Autodesk Fusion 360 part; units mm, degrees
(part 2 of 3)
sketch "Sketch6" plane through (0, 0, 6) normal (0, 0, 1) x (1, 0, 0)
  arc A0 (8.0454, -2.2316) -> (8.0834, -2.0901) centre (0, 0) ccw
  arc A1 (9.1959, -1.3509) -> (8.0834, -2.0901) centre (9.0515, -2.3404) ccw
  line L0 (9.1959, -1.3509) -> (9.7621, -1.4335)
  spline S0 degree 5 poles (9.7621, -1.4335) (9.7691, -1.4345) (9.783, -1.4364) (9.8041, -1.4384) (9.8322, -1.4399) (9.8676, -1.44) (9.903, -1.4389) (9.9385, -1.437) (9.9741, -1.4347) (10.0097, -1.4321) (10.0453, -1.4292) (10.081, -1.4258) (10.1167, -1.422) (10.1525, -1.4175) (10.1882, -1.4124) (10.224, -1.4067) (10.2599, -1.4005) (10.2957, -1.3939) (10.3316, -1.387) (10.3674, -1.3797) (10.4033, -1.3721) (10.4391, -1.364) (10.475, -1.3556) (10.5109, -1.3469) (10.5468, -1.3377) (10.5826, -1.3281) (10.6185, -1.3182) (10.6543, -1.3079) (10.6902, -1.2973) (10.726, -1.2864) (10.7619, -1.2752) (10.7977, -1.2636) (10.8335, -1.2517) (10.8693, -1.2395) (10.905, -1.227) (10.9408, -1.2141) (10.9765, -1.2009) (11.0122, -1.1875) (11.0479, -1.1737) (11.0835, -1.1597) (11.1191, -1.1453) (11.1547, -1.1307) (11.1903, -1.1158) (11.2259, -1.1005) (11.2614, -1.085) (11.2968, -1.0692) (11.3323, -1.0532) (11.3677, -1.0368) (11.4031, -1.0202) (11.4384, -1.0033) (11.4737, -0.9861) (11.5089, -0.9687) (11.5441, -0.951) (11.5793, -0.933) (11.6144, -0.9148) (11.6495, -0.8963) (11.6845, -0.8775) (11.7195, -0.8585) (11.7545, -0.8392) (11.7894, -0.8197) (11.8242, -0.7999) (11.859, -0.7799) (11.8937, -0.7596) (11.9284, -0.7391) (11.963, -0.7183) (11.9976, -0.6972) (12.0321, -0.6759) (12.0666, -0.6544) (12.101, -0.6327) (12.1353, -0.6106) (12.1696, -0.5884) (12.197, -0.5704) (12.2175, -0.5568) (12.2311, -0.5477) (12.238, -0.5431) knots 0 0 0 0 0 0 0.01428571 0.02857143 0.04285714 0.05714286 0.07142857 0.08571429 0.1 0.11428571 0.12857143 0.14285714 0.15714286 0.17142857 0.18571429 0.2 0.21428571 0.22857143 0.24285714 0.25714286 0.27142857 0.28571429 0.3 0.31428571 0.32857143 0.34285714 0.35714286 0.37142857 0.38571429 0.4 0.41428571 0.42857143 0.44285714 0.45714286 0.47142857 0.48571429 0.5 0.51428571 0.52857143 0.54285714 0.55714286 0.57142857 0.58571429 0.6 0.61428571 0.62857143 0.64285714 0.65714286 0.67142857 0.68571429 0.7 0.71428571 0.72857143 0.74285714 0.75714286 0.77142857 0.78571429 0.8 0.81428571 0.82857143 0.84285714 0.85714286 0.87142857 0.88571429 0.9 0.91428571 0.92857143 0.94285714 0.95714286 0.97142857 0.98571429 1 1 1 1 1 1
  arc A2 (12.238, -0.5431) -> (12.238, 0.5431) centre (0, 0) ccw
  spline S1 degree 5 poles (12.238, 0.5431) (12.2311, 0.5477) (12.2175, 0.5568) (12.197, 0.5704) (12.1696, 0.5884) (12.1353, 0.6106) (12.101, 0.6327) (12.0666, 0.6544) (12.0321, 0.6759) (11.9976, 0.6972) (11.963, 0.7183) (11.9284, 0.7391) (11.8937, 0.7596) (11.859, 0.7799) (11.8242, 0.7999) (11.7894, 0.8197) (11.7545, 0.8392) (11.7195, 0.8585) (11.6845, 0.8775) (11.6495, 0.8963) (11.6144, 0.9148) (11.5793, 0.933) (11.5441, 0.951) (11.5089, 0.9687) (11.4737, 0.9861) (11.4384, 1.0033) (11.4031, 1.0202) (11.3677, 1.0368) (11.3323, 1.0532) (11.2968, 1.0692) (11.2614, 1.085) (11.2259, 1.1005) (11.1903, 1.1158) (11.1547, 1.1307) (11.1191, 1.1453) (11.0835, 1.1597) (11.0479, 1.1737) (11.0122, 1.1875) (10.9765, 1.2009) (10.9408, 1.2141) (10.905, 1.227) (10.8693, 1.2395) (10.8335, 1.2517) (10.7977, 1.2636) (10.7619, 1.2752) (10.726, 1.2864) (10.6902, 1.2973) (10.6543, 1.3079) (10.6185, 1.3182) (10.5826, 1.3281) (10.5468, 1.3377) (10.5109, 1.3469) (10.475, 1.3556) (10.4391, 1.364) (10.4033, 1.3721) (10.3674, 1.3797) (10.3316, 1.387) (10.2957, 1.3939) (10.2599, 1.4005) (10.224, 1.4067) (10.1882, 1.4124) (10.1525, 1.4175) (10.1167, 1.422) (10.081, 1.4258) (10.0453, 1.4292) (10.0097, 1.4321) (9.9741, 1.4347) (9.9385, 1.437) (9.903, 1.4389) (9.8676, 1.44) (9.8322, 1.4399) (9.8041, 1.4384) (9.783, 1.4364) (9.7691, 1.4345) (9.7621, 1.4335) knots -1 -1 -1 -1 -1 -1 -0.98571429 -0.97142857 -0.95714286 -0.94285714 -0.92857143 -0.91428571 -0.9 -0.88571429 -0.87142857 -0.85714286 -0.84285714 -0.82857143 -0.81428571 -0.8 -0.78571429 -0.77142857 -0.75714286 -0.74285714 -0.72857143 -0.71428571 -0.7 -0.68571429 -0.67142857 -0.65714286 -0.64285714 -0.62857143 -0.61428571 -0.6 -0.58571429 -0.57142857 -0.55714286 -0.54285714 -0.52857143 -0.51428571 -0.5 -0.48571429 -0.47142857 -0.45714286 -0.44285714 -0.42857143 -0.41428571 -0.4 -0.38571429 -0.37142857 -0.35714286 -0.34285714 -0.32857143 -0.31428571 -0.3 -0.28571429 -0.27142857 -0.25714286 -0.24285714 -0.22857143 -0.21428571 -0.2 -0.18571429 -0.17142857 -0.15714286 -0.14285714 -0.12857143 -0.11428571 -0.1 -0.08571429 -0.07142857 -0.05714286 -0.04285714 -0.02857143 -0.01428571 0 0 0 0 0 0
  line L1 (9.7621, 1.4335) -> (9.1959, 1.3509)
  arc A3 (8.0834, 2.0901) -> (9.1959, 1.3509) centre (9.0515, 2.3404) ccw
  arc A4 (8.0834, 2.0901) -> (8.0454, 2.2316) centre (0, 0) ccw
  arc A5 (8.6393, 3.428) -> (8.0454, 2.2316) centre (9.0091, 2.4989) ccw
  line L2 (8.6393, 3.428) -> (9.171, 3.6396)
  spline S2 degree 5 poles (9.171, 3.6396) (9.1775, 3.6422) (9.1905, 3.6476) (9.2098, 3.6563) (9.2349, 3.6691) (9.2656, 3.6867) (9.2957, 3.7054) (9.3255, 3.7248) (9.3552, 3.7446) (9.3847, 3.7646) (9.4141, 3.785) (9.4433, 3.8057) (9.4723, 3.8269) (9.501, 3.8487) (9.5295, 3.871) (9.5576, 3.8938) (9.5856, 3.917) (9.6133, 3.9407) (9.6409, 3.9646) (9.6683, 3.9888) (9.6955, 4.0134) (9.7226, 4.0383) (9.7494, 4.0635) (9.7761, 4.089) (9.8026, 4.1149) (9.8289, 4.1411) (9.855, 4.1677) (9.8809, 4.1945) (9.9066, 4.2216) (9.9322, 4.249) (9.9576, 4.2766) (9.9829, 4.3045) (10.0079, 4.3327) (10.0328, 4.3612) (10.0575, 4.3899) (10.082, 4.4189) (10.1064, 4.4482) (10.1306, 4.4777) (10.1546, 4.5075) (10.1785, 4.5375) (10.2021, 4.5677) (10.2256, 4.5982) (10.249, 4.6289) (10.2721, 4.6598) (10.2951, 4.691) (10.318, 4.7224) (10.3406, 4.7541) (10.3631, 4.7859) (10.3854, 4.818) (10.4076, 4.8503) (10.4296, 4.8828) (10.4514, 4.9155) (10.473, 4.9485) (10.4945, 4.9816) (10.5158, 5.015) (10.5369, 5.0485) (10.5579, 5.0823) (10.5787, 5.1163) (10.5993, 5.1504) (10.6197, 5.1848) (10.64, 5.2193) (10.6601, 5.2541) (10.6801, 5.289) (10.6998, 5.3242) (10.7194, 5.3595) (10.7388, 5.395) (10.7581, 5.4307) (10.7772, 5.4665) (10.7961, 5.5026) (10.8148, 5.5388) (10.8334, 5.5752) (10.8481, 5.6045) (10.859, 5.6265) (10.8663, 5.6413) (10.8699, 5.6486) knots 0 0 0 0 0 0 0.01428571 0.02857143 0.04285714 0.05714286 0.07142857 0.08571429 0.1 0.11428571 0.12857143 0.14285714 0.15714286 0.17142857 0.18571429 0.2 0.21428571 0.22857143 0.24285714 0.25714286 0.27142857 0.28571429 0.3 0.31428571 0.32857143 0.34285714 0.35714286 0.37142857 0.38571429 0.4 0.41428571 0.42857143 0.44285714 0.45714286 0.47142857 0.48571429 0.5 0.51428571 0.52857143 0.54285714 0.55714286 0.57142857 0.58571429 0.6 0.61428571 0.62857143 0.64285714 0.65714286 0.67142857 0.68571429 0.7 0.71428571 0.72857143 0.74285714 0.75714286 0.77142857 0.78571429 0.8 0.81428571 0.82857143 0.84285714 0.85714286 0.87142857 0.88571429 0.9 0.91428571 0.92857143 0.94285714 0.95714286 0.97142857 0.98571429 1 1 1 1 1 1
  arc A6 (10.8699, 5.6486) -> (10.3268, 6.5893) centre (0, 0) ccw
  spline S3 degree 5 poles (10.3268, 6.5893) (10.3186, 6.5899) (10.3022, 6.5909) (10.2777, 6.5925) (10.245, 6.5944) (10.2042, 6.5965) (10.1634, 6.5984) (10.1228, 6.6) (10.0821, 6.6014) (10.0416, 6.6026) (10.0012, 6.6036) (9.9608, 6.6042) (9.9205, 6.6047) (9.8802, 6.6049) (9.8401, 6.6049) (9.8, 6.6046) (9.76, 6.604) (9.7202, 6.6033) (9.6803, 6.6022) (9.6406, 6.601) (9.601, 6.5994) (9.5615, 6.5977) (9.522, 6.5957) (9.4827, 6.5934) (9.4434, 6.5909) (9.4043, 6.5881) (9.3652, 6.585) (9.3263, 6.5818) (9.2875, 6.5782) (9.2487, 6.5744) (9.2101, 6.5703) (9.1716, 6.566) (9.1332, 6.5614) (9.095, 6.5566) (9.0568, 6.5515) (9.0188, 6.5461) (8.9809, 6.5404) (8.9431, 6.5345) (8.9054, 6.5283) (8.8679, 6.5218) (8.8305, 6.5151) (8.7933, 6.5081) (8.7562, 6.5007) (8.7193, 6.4931) (8.6825, 6.4852) (8.6458, 6.4771) (8.6093, 6.4686) (8.573, 6.4599) (8.5368, 6.4508) (8.5008, 6.4415) (8.4649, 6.4318) (8.4293, 6.4218) (8.3938, 6.4115) (8.3585, 6.4009) (8.3235, 6.3899) (8.2886, 6.3786) (8.2539, 6.367) (8.2194, 6.355) (8.185, 6.3428) (8.1509, 6.3303) (8.1171, 6.3173) (8.0836, 6.3038) (8.0504, 6.2898) (8.0175, 6.2753) (7.9849, 6.2604) (7.9526, 6.2451) (7.9205, 6.2295) (7.8885, 6.2138) (7.8568, 6.1976) (7.8255, 6.1809) (7.795, 6.1631) (7.7714, 6.1477) (7.7542, 6.1354) (7.743, 6.1269) (7.7374, 6.1225) knots -1 -1 -1 -1 -1 -1 -0.98571429 -0.97142857 -0.95714286 -0.94285714 -0.92857143 -0.91428571 -0.9 -0.88571429 -0.87142857 -0.85714286 -0.84285714 -0.82857143 -0.81428571 -0.8 -0.78571429 -0.77142857 -0.75714286 -0.74285714 -0.72857143 -0.71428571 -0.7 -0.68571429 -0.67142857 -0.65714286 -0.64285714 -0.62857143 -0.61428571 -0.6 -0.58571429 -0.57142857 -0.55714286 -0.54285714 -0.52857143 -0.51428571 -0.5 -0.48571429 -0.47142857 -0.45714286 -0.44285714 -0.42857143 -0.41428571 -0.4 -0.38571429 -0.37142857 -0.35714286 -0.34285714 -0.32857143 -0.31428571 -0.3 -0.28571429 -0.27142857 -0.25714286 -0.24285714 -0.22857143 -0.21428571 -0.2 -0.18571429 -0.17142857 -0.15714286 -0.14285714 -0.12857143 -0.11428571 -0.1 -0.08571429 -0.07142857 -0.05714286 -0.04285714 -0.02857143 -0.01428571 0 0 0 0 0 0
  line L3 (7.7374, 6.1225) -> (7.2884, 5.7679)
  arc A7 (5.9553, 5.8518) -> (7.2884, 5.7679) centre (6.6686, 6.5526) ccw
  arc A8 (5.9553, 5.8518) -> (5.8518, 5.9553) centre (0, 0) ccw
  arc A9 (5.7679, 7.2884) -> (5.8518, 5.9553) centre (6.5526, 6.6686) ccw
  line L4 (5.7679, 7.2884) -> (6.1225, 7.7374)
  spline S4 degree 5 poles (6.1225, 7.7374) (6.1269, 7.743) (6.1354, 7.7542) (6.1477, 7.7714) (6.1631, 7.795) (6.1809, 7.8255) (6.1976, 7.8568) (6.2138, 7.8885) (6.2295, 7.9205) (6.2451, 7.9526) (6.2604, 7.9849) (6.2753, 8.0175) (6.2898, 8.0504) (6.3038, 8.0836) (6.3173, 8.1171) (6.3303, 8.1509) (6.3428, 8.185) (6.355, 8.2194) (6.367, 8.2539) (6.3786, 8.2886) (6.3899, 8.3235) (6.4009, 8.3585) (6.4115, 8.3938) (6.4218, 8.4293) (6.4318, 8.4649) (6.4415, 8.5008) (6.4508, 8.5368) (6.4599, 8.573) (6.4686, 8.6093) (6.4771, 8.6458) (6.4852, 8.6825) (6.4931, 8.7193) (6.5007, 8.7562) (6.5081, 8.7933) (6.5151, 8.8305) (6.5218, 8.8679) (6.5283, 8.9054) (6.5345, 8.9431) (6.5404, 8.9809) (6.5461, 9.0188) (6.5515, 9.0568) (6.5566, 9.095) (6.5614, 9.1332) (6.566, 9.1716) (6.5703, 9.2101) (6.5744, 9.2487) (6.5782, 9.2875) (6.5818, 9.3263) (6.585, 9.3652) (6.5881, 9.4043) (6.5909, 9.4434) (6.5934, 9.4827) (6.5957, 9.522) (6.5977, 9.5615) (6.5994, 9.601) (6.601, 9.6406) (6.6022, 9.6803) (6.6033, 9.7202) (6.604, 9.76) (6.6046, 9.8) (6.6049, 9.8401) (6.6049, 9.8802) (6.6047, 9.9205) (6.6042, 9.9608) (6.6036, 10.0012) (6.6026, 10.0416) (6.6014, 10.0821) (6.6, 10.1228) (6.5984, 10.1634) (6.5965, 10.2042) (6.5944, 10.245) (6.5925, 10.2777) (6.5909, 10.3022) (6.5899, 10.3186) (6.5893, 10.3268) knots 0 0 0 0 0 0 0.01428571 0.02857143 0.04285714 0.05714286 0.07142857 0.08571429 0.1 0.11428571 0.12857143 0.14285714 0.15714286 0.17142857 0.18571429 0.2 0.21428571 0.22857143 0.24285714 0.25714286 0.27142857 0.28571429 0.3 0.31428571 0.32857143 0.34285714 0.35714286 0.37142857 0.38571429 0.4 0.41428571 0.42857143 0.44285714 0.45714286 0.47142857 0.48571429 0.5 0.51428571 0.52857143 0.54285714 0.55714286 0.57142857 0.58571429 0.6 0.61428571 0.62857143 0.64285714 0.65714286 0.67142857 0.68571429 0.7 0.71428571 0.72857143 0.74285714 0.75714286 0.77142857 0.78571429 0.8 0.81428571 0.82857143 0.84285714 0.85714286 0.87142857 0.88571429 0.9 0.91428571 0.92857143 0.94285714 0.95714286 0.97142857 0.98571429 1 1 1 1 1 1
  arc A10 (6.5893, 10.3268) -> (5.6486, 10.8699) centre (0, 0) ccw
  spline S5 degree 5 poles (5.6486, 10.8699) (5.6413, 10.8663) (5.6265, 10.859) (5.6045, 10.8481) (5.5752, 10.8334) (5.5388, 10.8148) (5.5026, 10.7961) (5.4665, 10.7772) (5.4307, 10.7581) (5.395, 10.7388) (5.3595, 10.7194) (5.3242, 10.6998) (5.289, 10.6801) (5.2541, 10.6601) (5.2193, 10.64) (5.1848, 10.6197) (5.1504, 10.5993) (5.1163, 10.5787) (5.0823, 10.5579) (5.0485, 10.5369) (5.015, 10.5158) (4.9816, 10.4945) (4.9485, 10.473) (4.9155, 10.4514) (4.8828, 10.4296) (4.8503, 10.4076) (4.818, 10.3854) (4.7859, 10.3631) (4.7541, 10.3406) (4.7224, 10.318) (4.691, 10.2951) (4.6598, 10.2721) (4.6289, 10.249) (4.5982, 10.2256) (4.5677, 10.2021) (4.5375, 10.1785) (4.5075, 10.1546) (4.4777, 10.1306) (4.4482, 10.1064) (4.4189, 10.082) (4.3899, 10.0575) (4.3612, 10.0328) (4.3327, 10.0079) (4.3045, 9.9829) (4.2766, 9.9576) (4.249, 9.9322) (4.2216, 9.9066) (4.1945, 9.8809) (4.1677, 9.855) (4.1411, 9.8289) (4.1149, 9.8026) (4.089, 9.7761) (4.0635, 9.7494) (4.0383, 9.7226) (4.0134, 9.6955) (3.9888, 9.6683) (3.9646, 9.6409) (3.9407, 9.6133) (3.917, 9.5856) (3.8938, 9.5576) (3.871, 9.5295) (3.8487, 9.501) (3.8269, 9.4723) (3.8057, 9.4433) (3.785, 9.4141) (3.7646, 9.3847) (3.7446, 9.3552) (3.7248, 9.3255) (3.7054, 9.2957) (3.6867, 9.2656) (3.6691, 9.2349) (3.6563, 9.2098) (3.6476, 9.1905) (3.6422, 9.1775) (3.6396, 9.171) knots -1 -1 -1 -1 -1 -1 -0.98571429 -0.97142857 -0.95714286 -0.94285714 -0.92857143 -0.91428571 -0.9 -0.88571429 -0.87142857 -0.85714286 -0.84285714 -0.82857143 -0.81428571 -0.8 -0.78571429 -0.77142857 -0.75714286 -0.74285714 -0.72857143 -0.71428571 -0.7 -0.68571429 -0.67142857 -0.65714286 -0.64285714 -0.62857143 -0.61428571 -0.6 -0.58571429 -0.57142857 -0.55714286 -0.54285714 -0.52857143 -0.51428571 -0.5 -0.48571429 -0.47142857 -0.45714286 -0.44285714 -0.42857143 -0.41428571 -0.4 -0.38571429 -0.37142857 -0.35714286 -0.34285714 -0.32857143 -0.31428571 -0.3 -0.28571429 -0.27142857 -0.25714286 -0.24285714 -0.22857143 -0.21428571 -0.2 -0.18571429 -0.17142857 -0.15714286 -0.14285714 -0.12857143 -0.11428571 -0.1 -0.08571429 -0.07142857 -0.05714286 -0.04285714 -0.02857143 -0.01428571 0 0 0 0 0 0
  line L5 (3.6396, 9.171) -> (3.428, 8.6393)
  arc A11 (2.2316, 8.0454) -> (3.428, 8.6393) centre (2.4989, 9.0091) ccw
  arc A12 (2.2316, 8.0454) -> (2.0901, 8.0834) centre (0, 0) ccw
  arc A13 (1.3509, 9.1959) -> (2.0901, 8.0834) centre (2.3404, 9.0515) ccw
  line L6 (1.3509, 9.1959) -> (1.4335, 9.7621)
  spline S6 degree 5 poles (1.4335, 9.7621) (1.4345, 9.7691) (1.4364, 9.783) (1.4384, 9.8041) (1.4399, 9.8322) (1.44, 9.8676) (1.4389, 9.903) (1.437, 9.9385) (1.4347, 9.9741) (1.4321, 10.0097) (1.4292, 10.0453) (1.4258, 10.081) (1.422, 10.1167) (1.4175, 10.1525) (1.4124, 10.1882) (1.4067, 10.224) (1.4005, 10.2599) (1.3939, 10.2957) (1.387, 10.3316) (1.3797, 10.3674) (1.3721, 10.4033) (1.364, 10.4391) (1.3556, 10.475) (1.3469, 10.5109) (1.3377, 10.5468) (1.3281, 10.5826) (1.3182, 10.6185) (1.3079, 10.6543) (1.2973, 10.6902) (1.2864, 10.726) (1.2752, 10.7619) (1.2636, 10.7977) (1.2517, 10.8335) (1.2395, 10.8693) (1.227, 10.905) (1.2141, 10.9408) (1.2009, 10.9765) (1.1875, 11.0122) (1.1737, 11.0479) (1.1597, 11.0835) (1.1453, 11.1191) (1.1307, 11.1547) (1.1158, 11.1903) (1.1005, 11.2259) (1.085, 11.2614) (1.0692, 11.2968) (1.0532, 11.3323) (1.0368, 11.3677) (1.0202, 11.4031) (1.0033, 11.4384) (0.9861, 11.4737) (0.9687, 11.5089) (0.951, 11.5441) (0.933, 11.5793) (0.9148, 11.6144) (0.8963, 11.6495) (0.8775, 11.6845) (0.8585, 11.7195) (0.8392, 11.7545) (0.8197, 11.7894) (0.7999, 11.8242) (0.7799, 11.859) (0.7596, 11.8937) (0.7391, 11.9284) (0.7183, 11.963) (0.6972, 11.9976) (0.6759, 12.0321) (0.6544, 12.0666) (0.6327, 12.101) (0.6106, 12.1353) (0.5884, 12.1696) (0.5704, 12.197) (0.5568, 12.2175) (0.5477, 12.2311) (0.5431, 12.238) knots 0 0 0 0 0 0 0.01428571 0.02857143 0.04285714 0.05714286 0.07142857 0.08571429 0.1 0.11428571 0.12857143 0.14285714 0.15714286 0.17142857 0.18571429 0.2 0.21428571 0.22857143 0.24285714 0.25714286 0.27142857 0.28571429 0.3 0.31428571 0.32857143 0.34285714 0.35714286 0.37142857 0.38571429 0.4 0.41428571 0.42857143 0.44285714 0.45714286 0.47142857 0.48571429 0.5 0.51428571 0.52857143 0.54285714 0.55714286 0.57142857 0.58571429 0.6 0.61428571 0.62857143 0.64285714 0.65714286 0.67142857 0.68571429 0.7 0.71428571 0.72857143 0.74285714 0.75714286 0.77142857 0.78571429 0.8 0.81428571 0.82857143 0.84285714 0.85714286 0.87142857 0.88571429 0.9 0.91428571 0.92857143 0.94285714 0.95714286 0.97142857 0.98571429 1 1 1 1 1 1
  arc A14 (0.5431, 12.238) -> (-0.5431, 12.238) centre (0, 0) ccw
  spline S7 degree 5 poles (-0.5431, 12.238) (-0.5477, 12.2311) (-0.5568, 12.2175) (-0.5704, 12.197) (-0.5884, 12.1696) (-0.6106, 12.1353) (-0.6327, 12.101) (-0.6544, 12.0666) (-0.6759, 12.0321) (-0.6972, 11.9976) (-0.7183, 11.963) (-0.7391, 11.9284) (-0.7596, 11.8937) (-0.7799, 11.859) (-0.7999, 11.8242) (-0.8197, 11.7894) (-0.8392, 11.7545) (-0.8585, 11.7195) (-0.8775, 11.6845) (-0.8963, 11.6495) (-0.9148, 11.6144) (-0.933, 11.5793) (-0.951, 11.5441) (-0.9687, 11.5089) (-0.9861, 11.4737) (-1.0033, 11.4384) (-1.0202, 11.4031) (-1.0368, 11.3677) (-1.0532, 11.3323) (-1.0692, 11.2968) (-1.085, 11.2614) (-1.1005, 11.2259) (-1.1158, 11.1903) (-1.1307, 11.1547) (-1.1453, 11.1191) (-1.1597, 11.0835) (-1.1737, 11.0479) (-1.1875, 11.0122) (-1.2009, 10.9765) (-1.2141, 10.9408) (-1.227, 10.905) (-1.2395, 10.8693) (-1.2517, 10.8335) (-1.2636, 10.7977) (-1.2752, 10.7619) (-1.2864, 10.726) (-1.2973, 10.6902) (-1.3079, 10.6543) (-1.3182, 10.6185) (-1.3281, 10.5826) (-1.3377, 10.5468) (-1.3469, 10.5109) (-1.3556, 10.475) (-1.364, 10.4391) (-1.3721, 10.4033) (-1.3797, 10.3674) (-1.387, 10.3316) (-1.3939, 10.2957) (-1.4005, 10.2599) (-1.4067, 10.224) (-1.4124, 10.1882) (-1.4175, 10.1525) (-1.422, 10.1167) (-1.4258, 10.081) (-1.4292, 10.0453) (-1.4321, 10.0097) (-1.4347, 9.9741) (-1.437, 9.9385) (-1.4389, 9.903) (-1.44, 9.8676) (-1.4399, 9.8322) (-1.4384, 9.8041) (-1.4364, 9.783) (-1.4345, 9.7691) (-1.4335, 9.7621) knots -1 -1 -1 -1 -1 -1 -0.98571429 -0.97142857 -0.95714286 -0.94285714 -0.92857143 -0.91428571 -0.9 -0.88571429 -0.87142857 -0.85714286 -0.84285714 -0.82857143 -0.81428571 -0.8 -0.78571429 -0.77142857 -0.75714286 -0.74285714 -0.72857143 -0.71428571 -0.7 -0.68571429 -0.67142857 -0.65714286 -0.64285714 -0.62857143 -0.61428571 -0.6 -0.58571429 -0.57142857 -0.55714286 -0.54285714 -0.52857143 -0.51428571 -0.5 -0.48571429 -0.47142857 -0.45714286 -0.44285714 -0.42857143 -0.41428571 -0.4 -0.38571429 -0.37142857 -0.35714286 -0.34285714 -0.32857143 -0.31428571 -0.3 -0.28571429 -0.27142857 -0.25714286 -0.24285714 -0.22857143 -0.21428571 -0.2 -0.18571429 -0.17142857 -0.15714286 -0.14285714 -0.12857143 -0.11428571 -0.1 -0.08571429 -0.07142857 -0.05714286 -0.04285714 -0.02857143 -0.01428571 0 0 0 0 0 0
  line L7 (-1.4335, 9.7621) -> (-1.3509, 9.1959)
  arc A15 (-2.0901, 8.0834) -> (-1.3509, 9.1959) centre (-2.3404, 9.0515) ccw
  arc A16 (-2.0901, 8.0834) -> (-2.2316, 8.0454) centre (0, 0) ccw
  arc A17 (-3.428, 8.6393) -> (-2.2316, 8.0454) centre (-2.4989, 9.0091) ccw
  line L8 (-3.428, 8.6393) -> (-3.6396, 9.171)
  spline S8 degree 5 poles (-3.6396, 9.171) (-3.6422, 9.1775) (-3.6476, 9.1905) (-3.6563, 9.2098) (-3.6691, 9.2349) (-3.6867, 9.2656) (-3.7054, 9.2957) (-3.7248, 9.3255) (-3.7446, 9.3552) (-3.7646, 9.3847) (-3.785, 9.4141) (-3.8057, 9.4433) (-3.8269, 9.4723) (-3.8487, 9.501) (-3.871, 9.5295) (-3.8938, 9.5576) (-3.917, 9.5856) (-3.9407, 9.6133) (-3.9646, 9.6409) (-3.9888, 9.6683) (-4.0134, 9.6955) (-4.0383, 9.7226) (-4.0635, 9.7494) (-4.089, 9.7761) (-4.1149, 9.8026) (-4.1411, 9.8289) (-4.1677, 9.855) (-4.1945, 9.8809) (-4.2216, 9.9066) (-4.249, 9.9322) (-4.2766, 9.9576) (-4.3045, 9.9829) (-4.3327, 10.0079) (-4.3612, 10.0328) (-4.3899, 10.0575) (-4.4189, 10.082) (-4.4482, 10.1064) (-4.4777, 10.1306) (-4.5075, 10.1546) (-4.5375, 10.1785) (-4.5677, 10.2021) (-4.5982, 10.2256) (-4.6289, 10.249) (-4.6598, 10.2721) (-4.691, 10.2951) (-4.7224, 10.318) (-4.7541, 10.3406) (-4.7859, 10.3631) (-4.818, 10.3854) (-4.8503, 10.4076) (-4.8828, 10.4296) (-4.9155, 10.4514) (-4.9485, 10.473) (-4.9816, 10.4945) (-5.015, 10.5158) (-5.0485, 10.5369) (-5.0823, 10.5579) (-5.1163, 10.5787) (-5.1504, 10.5993) (-5.1848, 10.6197) (-5.2193, 10.64) (-5.2541, 10.6601) (-5.289, 10.6801) (-5.3242, 10.6998) (-5.3595, 10.7194) (-5.395, 10.7388) (-5.4307, 10.7581) (-5.4665, 10.7772) (-5.5026, 10.7961) (-5.5388, 10.8148) (-5.5752, 10.8334) (-5.6045, 10.8481) (-5.6265, 10.859) (-5.6413, 10.8663) (-5.6486, 10.8699) knots 0 0 0 0 0 0 0.01428571 0.02857143 0.04285714 0.05714286 0.07142857 0.08571429 0.1 0.11428571 0.12857143 0.14285714 0.15714286 0.17142857 0.18571429 0.2 0.21428571 0.22857143 0.24285714 0.25714286 0.27142857 0.28571429 0.3 0.31428571 0.32857143 0.34285714 0.35714286 0.37142857 0.38571429 0.4 0.41428571 0.42857143 0.44285714 0.45714286 0.47142857 0.48571429 0.5 0.51428571 0.52857143 0.54285714 0.55714286 0.57142857 0.58571429 0.6 0.61428571 0.62857143 0.64285714 0.65714286 0.67142857 0.68571429 0.7 0.71428571 0.72857143 0.74285714 0.75714286 0.77142857 0.78571429 0.8 0.81428571 0.82857143 0.84285714 0.85714286 0.87142857 0.88571429 0.9 0.91428571 0.92857143 0.94285714 0.95714286 0.97142857 0.98571429 1 1 1 1 1 1
  arc A18 (-5.6486, 10.8699) -> (-6.5893, 10.3268) centre (0, 0) ccw
  spline S9 degree 5 poles (-6.5893, 10.3268) (-6.5899, 10.3186) (-6.5909, 10.3022) (-6.5925, 10.2777) (-6.5944, 10.245) (-6.5965, 10.2042) (-6.5984, 10.1634) (-6.6, 10.1228) (-6.6014, 10.0821) (-6.6026, 10.0416) (-6.6036, 10.0012) (-6.6042, 9.9608) (-6.6047, 9.9205) (-6.6049, 9.8802) (-6.6049, 9.8401) (-6.6046, 9.8) (-6.604, 9.76) (-6.6033, 9.7202) (-6.6022, 9.6803) (-6.601, 9.6406) (-6.5994, 9.601) (-6.5977, 9.5615) (-6.5957, 9.522) (-6.5934, 9.4827) (-6.5909, 9.4434) (-6.5881, 9.4043) (-6.585, 9.3652) (-6.5818, 9.3263) (-6.5782, 9.2875) (-6.5744, 9.2487) (-6.5703, 9.2101) (-6.566, 9.1716) (-6.5614, 9.1332) (-6.5566, 9.095) (-6.5515, 9.0568) (-6.5461, 9.0188) (-6.5404, 8.9809) (-6.5345, 8.9431) (-6.5283, 8.9054) (-6.5218, 8.8679) (-6.5151, 8.8305) (-6.5081, 8.7933) (-6.5007, 8.7562) (-6.4931, 8.7193) (-6.4852, 8.6825) (-6.4771, 8.6458) (-6.4686, 8.6093) (-6.4599, 8.573) (-6.4508, 8.5368) (-6.4415, 8.5008) (-6.4318, 8.4649) (-6.4218, 8.4293) (-6.4115, 8.3938) (-6.4009, 8.3585) (-6.3899, 8.3235) (-6.3786, 8.2886) (-6.367, 8.2539) (-6.355, 8.2194) (-6.3428, 8.185) (-6.3303, 8.1509) (-6.3173, 8.1171) (-6.3038, 8.0836) (-6.2898, 8.0504) (-6.2753, 8.0175) (-6.2604, 7.9849) (-6.2451, 7.9526) (-6.2295, 7.9205) (-6.2138, 7.8885) (-6.1976, 7.8568) (-6.1809, 7.8255) (-6.1631, 7.795) (-6.1477, 7.7714) (-6.1354, 7.7542) (-6.1269, 7.743) (-6.1225, 7.7374) knots -1 -1 -1 -1 -1 -1 -0.98571429 -0.97142857 -0.95714286 -0.94285714 -0.92857143 -0.91428571 -0.9 -0.88571429 -0.87142857 -0.85714286 -0.84285714 -0.82857143 -0.81428571 -0.8 -0.78571429 -0.77142857 -0.75714286 -0.74285714 -0.72857143 -0.71428571 -0.7 -0.68571429 -0.67142857 -0.65714286 -0.64285714 -0.62857143 -0.61428571 -0.6 -0.58571429 -0.57142857 -0.55714286 -0.54285714 -0.52857143 -0.51428571 -0.5 -0.48571429 -0.47142857 -0.45714286 -0.44285714 -0.42857143 -0.41428571 -0.4 -0.38571429 -0.37142857 -0.35714286 -0.34285714 -0.32857143 -0.31428571 -0.3 -0.28571429 -0.27142857 -0.25714286 -0.24285714 -0.22857143 -0.21428571 -0.2 -0.18571429 -0.17142857 -0.15714286 -0.14285714 -0.12857143 -0.11428571 -0.1 -0.08571429 -0.07142857 -0.05714286 -0.04285714 -0.02857143 -0.01428571 0 0 0 0 0 0
  line L9 (-6.1225, 7.7374) -> (-5.7679, 7.2884)
  arc A19 (-5.8518, 5.9553) -> (-5.7679, 7.2884) centre (-6.5526, 6.6686) ccw
  arc A20 (-5.8518, 5.9553) -> (-5.9553, 5.8518) centre (0, 0) ccw
  arc A21 (-7.2884, 5.7679) -> (-5.9553, 5.8518) centre (-6.6686, 6.5526) ccw
  line L10 (-7.2884, 5.7679) -> (-7.7374, 6.1225)
  spline S10 degree 5 poles (-7.7374, 6.1225) (-7.743, 6.1269) (-7.7542, 6.1354) (-7.7714, 6.1477) (-7.795, 6.1631) (-7.8255, 6.1809) (-7.8568, 6.1976) (-7.8885, 6.2138) (-7.9205, 6.2295) (-7.9526, 6.2451) (-7.9849, 6.2604) (-8.0175, 6.2753) (-8.0504, 6.2898) (-8.0836, 6.3038) (-8.1171, 6.3173) (-8.1509, 6.3303) (-8.185, 6.3428) (-8.2194, 6.355) (-8.2539, 6.367) (-8.2886, 6.3786) (-8.3235, 6.3899) (-8.3585, 6.4009) (-8.3938, 6.4115) (-8.4293, 6.4218) (-8.4649, 6.4318) (-8.5008, 6.4415) (-8.5368, 6.4508) (-8.573, 6.4599) (-8.6093, 6.4686) (-8.6458, 6.4771) (-8.6825, 6.4852) (-8.7193, 6.4931) (-8.7562, 6.5007) (-8.7933, 6.5081) (-8.8305, 6.5151) (-8.8679, 6.5218) (-8.9054, 6.5283) (-8.9431, 6.5345) (-8.9809, 6.5404) (-9.0188, 6.5461) (-9.0568, 6.5515) (-9.095, 6.5566) (-9.1332, 6.5614) (-9.1716, 6.566) (-9.2101, 6.5703) (-9.2487, 6.5744) (-9.2875, 6.5782) (-9.3263, 6.5818) (-9.3652, 6.585) (-9.4043, 6.5881) (-9.4434, 6.5909) (-9.4827, 6.5934) (-9.522, 6.5957) (-9.5615, 6.5977) (-9.601, 6.5994) (-9.6406, 6.601) (-9.6803, 6.6022) (-9.7202, 6.6033) (-9.76, 6.604) (-9.8, 6.6046) (-9.8401, 6.6049) (-9.8802, 6.6049) (-9.9205, 6.6047) (-9.9608, 6.6042) (-10.0012, 6.6036) (-10.0416, 6.6026) (-10.0821, 6.6014) (-10.1228, 6.6) (-10.1634, 6.5984) (-10.2042, 6.5965) (-10.245, 6.5944) (-10.2777, 6.5925) (-10.3022, 6.5909) (-10.3186, 6.5899) (-10.3268, 6.5893) knots 0 0 0 0 0 0 0.01428571 0.02857143 0.04285714 0.05714286 0.07142857 0.08571429 0.1 0.11428571 0.12857143 0.14285714 0.15714286 0.17142857 0.18571429 0.2 0.21428571 0.22857143 0.24285714 0.25714286 0.27142857 0.28571429 0.3 0.31428571 0.32857143 0.34285714 0.35714286 0.37142857 0.38571429 0.4 0.41428571 0.42857143 0.44285714 0.45714286 0.47142857 0.48571429 0.5 0.51428571 0.52857143 0.54285714 0.55714286 0.57142857 0.58571429 0.6 0.61428571 0.62857143 0.64285714 0.65714286 0.67142857 0.68571429 0.7 0.71428571 0.72857143 0.74285714 0.75714286 0.77142857 0.78571429 0.8 0.81428571 0.82857143 0.84285714 0.85714286 0.87142857 0.88571429 0.9 0.91428571 0.92857143 0.94285714 0.95714286 0.97142857 0.98571429 1 1 1 1 1 1
  arc A22 (-10.3268, 6.5893) -> (-10.8699, 5.6486) centre (0, 0) ccw
  spline S11 degree 5 poles (-10.8699, 5.6486) (-10.8663, 5.6413) (-10.859, 5.6265) (-10.8481, 5.6045) (-10.8334, 5.5752) (-10.8148, 5.5388) (-10.7961, 5.5026) (-10.7772, 5.4665) (-10.7581, 5.4307) (-10.7388, 5.395) (-10.7194, 5.3595) (-10.6998, 5.3242) (-10.6801, 5.289) (-10.6601, 5.2541) (-10.64, 5.2193) (-10.6197, 5.1848) (-10.5993, 5.1504) (-10.5787, 5.1163) (-10.5579, 5.0823) (-10.5369, 5.0485) (-10.5158, 5.015) (-10.4945, 4.9816) (-10.473, 4.9485) (-10.4514, 4.9155) (-10.4296, 4.8828) (-10.4076, 4.8503) (-10.3854, 4.818) (-10.3631, 4.7859) (-10.3406, 4.7541) (-10.318, 4.7224) (-10.2951, 4.691) (-10.2721, 4.6598) (-10.249, 4.6289) (-10.2256, 4.5982) (-10.2021, 4.5677) (-10.1785, 4.5375) (-10.1546, 4.5075) (-10.1306, 4.4777) (-10.1064, 4.4482) (-10.082, 4.4189) (-10.0575, 4.3899) (-10.0328, 4.3612) (-10.0079, 4.3327) (-9.9829, 4.3045) (-9.9576, 4.2766) (-9.9322, 4.249) (-9.9066, 4.2216) (-9.8809, 4.1945) (-9.855, 4.1677) (-9.8289, 4.1411) (-9.8026, 4.1149) (-9.7761, 4.089) (-9.7494, 4.0635) (-9.7226, 4.0383) (-9.6955, 4.0134) (-9.6683, 3.9888) (-9.6409, 3.9646) (-9.6133, 3.9407) (-9.5856, 3.917) (-9.5576, 3.8938) (-9.5295, 3.871) (-9.501, 3.8487) (-9.4723, 3.8269) (-9.4433, 3.8057) (-9.4141, 3.785) (-9.3847, 3.7646) (-9.3552, 3.7446) (-9.3255, 3.7248) (-9.2957, 3.7054) (-9.2656, 3.6867) (-9.2349, 3.6691) (-9.2098, 3.6563) (-9.1905, 3.6476) (-9.1775, 3.6422) (-9.171, 3.6396) knots -1 -1 -1 -1 -1 -1 -0.98571429 -0.97142857 -0.95714286 -0.94285714 -0.92857143 -0.91428571 -0.9 -0.88571429 -0.87142857 -0.85714286 -0.84285714 -0.82857143 -0.81428571 -0.8 -0.78571429 -0.77142857 -0.75714286 -0.74285714 -0.72857143 -0.71428571 -0.7 -0.68571429 -0.67142857 -0.65714286 -0.64285714 -0.62857143 -0.61428571 -0.6 -0.58571429 -0.57142857 -0.55714286 -0.54285714 -0.52857143 -0.51428571 -0.5 -0.48571429 -0.47142857 -0.45714286 -0.44285714 -0.42857143 -0.41428571 -0.4 -0.38571429 -0.37142857 -0.35714286 -0.34285714 -0.32857143 -0.31428571 -0.3 -0.28571429 -0.27142857 -0.25714286 -0.24285714 -0.22857143 -0.21428571 -0.2 -0.18571429 -0.17142857 -0.15714286 -0.14285714 -0.12857143 -0.11428571 -0.1 -0.08571429 -0.07142857 -0.05714286 -0.04285714 -0.02857143 -0.01428571 0 0 0 0 0 0
  line L11 (-9.171, 3.6396) -> (-8.6393, 3.428)
  arc A23 (-8.0454, 2.2316) -> (-8.6393, 3.428) centre (-9.0091, 2.4989) ccw
  arc A24 (-8.0454, 2.2316) -> (-8.0834, 2.0901) centre (0, 0) ccw
  arc A25 (-9.1959, 1.3509) -> (-8.0834, 2.0901) centre (-9.0515, 2.3404) ccw
  line L12 (-9.1959, 1.3509) -> (-9.7621, 1.4335)
  spline S12 degree 5 poles (-9.7621, 1.4335) (-9.7691, 1.4345) (-9.783, 1.4364) (-9.8041, 1.4384) (-9.8322, 1.4399) (-9.8676, 1.44) (-9.903, 1.4389) (-9.9385, 1.437) (-9.9741, 1.4347) (-10.0097, 1.4321) (-10.0453, 1.4292) (-10.081, 1.4258) (-10.1167, 1.422) (-10.1525, 1.4175) (-10.1882, 1.4124) (-10.224, 1.4067) (-10.2599, 1.4005) (-10.2957, 1.3939) (-10.3316, 1.387) (-10.3674, 1.3797) (-10.4033, 1.3721) (-10.4391, 1.364) (-10.475, 1.3556) (-10.5109, 1.3469) (-10.5468, 1.3377) (-10.5826, 1.3281) (-10.6185, 1.3182) (-10.6543, 1.3079) (-10.6902, 1.2973) (-10.726, 1.2864) (-10.7619, 1.2752) (-10.7977, 1.2636) (-10.8335, 1.2517) (-10.8693, 1.2395) (-10.905, 1.227) (-10.9408, 1.2141) (-10.9765, 1.2009) (-11.0122, 1.1875) (-11.0479, 1.1737) (-11.0835, 1.1597) (-11.1191, 1.1453) (-11.1547, 1.1307) (-11.1903, 1.1158) (-11.2259, 1.1005) (-11.2614, 1.085) (-11.2968, 1.0692) (-11.3323, 1.0532) (-11.3677, 1.0368) (-11.4031, 1.0202) (-11.4384, 1.0033) (-11.4737, 0.9861) (-11.5089, 0.9687) (-11.5441, 0.951) (-11.5793, 0.933) (-11.6144, 0.9148) (-11.6495, 0.8963) (-11.6845, 0.8775) (-11.7195, 0.8585) (-11.7545, 0.8392) (-11.7894, 0.8197) (-11.8242, 0.7999) (-11.859, 0.7799) (-11.8937, 0.7596) (-11.9284, 0.7391) (-11.963, 0.7183) (-11.9976, 0.6972) (-12.0321, 0.6759) (-12.0666, 0.6544) (-12.101, 0.6327) (-12.1353, 0.6106) (-12.1696, 0.5884) (-12.197, 0.5704) (-12.2175, 0.5568) (-12.2311, 0.5477) (-12.238, 0.5431) knots 0 0 0 0 0 0 0.01428571 0.02857143 0.04285714 0.05714286 0.07142857 0.08571429 0.1 0.11428571 0.12857143 0.14285714 0.15714286 0.17142857 0.18571429 0.2 0.21428571 0.22857143 0.24285714 0.25714286 0.27142857 0.28571429 0.3 0.31428571 0.32857143 0.34285714 0.35714286 0.37142857 0.38571429 0.4 0.41428571 0.42857143 0.44285714 0.45714286 0.47142857 0.48571429 0.5 0.51428571 0.52857143 0.54285714 0.55714286 0.57142857 0.58571429 0.6 0.61428571 0.62857143 0.64285714 0.65714286 0.67142857 0.68571429 0.7 0.71428571 0.72857143 0.74285714 0.75714286 0.77142857 0.78571429 0.8 0.81428571 0.82857143 0.84285714 0.85714286 0.87142857 0.88571429 0.9 0.91428571 0.92857143 0.94285714 0.95714286 0.97142857 0.98571429 1 1 1 1 1 1
  arc A26 (-12.238, 0.5431) -> (-12.238, -0.5431) centre (0, 0) ccw
  spline S13 degree 5 poles (-12.238, -0.5431) (-12.2311, -0.5477) (-12.2175, -0.5568) (-12.197, -0.5704) (-12.1696, -0.5884) (-12.1353, -0.6106) (-12.101, -0.6327) (-12.0666, -0.6544) (-12.0321, -0.6759) (-11.9976, -0.6972) (-11.963, -0.7183) (-11.9284, -0.7391) (-11.8937, -0.7596) (-11.859, -0.7799) (-11.8242, -0.7999) (-11.7894, -0.8197) (-11.7545, -0.8392) (-11.7195, -0.8585) (-11.6845, -0.8775) (-11.6495, -0.8963) (-11.6144, -0.9148) (-11.5793, -0.933) (-11.5441, -0.951) (-11.5089, -0.9687) (-11.4737, -0.9861) (-11.4384, -1.0033) (-11.4031, -1.0202) (-11.3677, -1.0368) (-11.3323, -1.0532) (-11.2968, -1.0692) (-11.2614, -1.085) (-11.2259, -1.1005) (-11.1903, -1.1158) (-11.1547, -1.1307) (-11.1191, -1.1453) (-11.0835, -1.1597) (-11.0479, -1.1737) (-11.0122, -1.1875) (-10.9765, -1.2009) (-10.9408, -1.2141) (-10.905, -1.227) (-10.8693, -1.2395) (-10.8335, -1.2517) (-10.7977, -1.2636) (-10.7619, -1.2752) (-10.726, -1.2864) (-10.6902, -1.2973) (-10.6543, -1.3079) (-10.6185, -1.3182) (-10.5826, -1.3281) (-10.5468, -1.3377) (-10.5109, -1.3469) (-10.475, -1.3556) (-10.4391, -1.364) (-10.4033, -1.3721) (-10.3674, -1.3797) (-10.3316, -1.387) (-10.2957, -1.3939) (-10.2599, -1.4005) (-10.224, -1.4067) (-10.1882, -1.4124) (-10.1525, -1.4175) (-10.1167, -1.422) (-10.081, -1.4258) (-10.0453, -1.4292) (-10.0097, -1.4321) (-9.9741, -1.4347) (-9.9385, -1.437) (-9.903, -1.4389) (-9.8676, -1.44) (-9.8322, -1.4399) (-9.8041, -1.4384) (-9.783, -1.4364) (-9.7691, -1.4345) (-9.7621, -1.4335) knots -1 -1 -1 -1 -1 -1 -0.98571429 -0.97142857 -0.95714286 -0.94285714 -0.92857143 -0.91428571 -0.9 -0.88571429 -0.87142857 -0.85714286 -0.84285714 -0.82857143 -0.81428571 -0.8 -0.78571429 -0.77142857 -0.75714286 -0.74285714 -0.72857143 -0.71428571 -0.7 -0.68571429 -0.67142857 -0.65714286 -0.64285714 -0.62857143 -0.61428571 -0.6 -0.58571429 -0.57142857 -0.55714286 -0.54285714 -0.52857143 -0.51428571 -0.5 -0.48571429 -0.47142857 -0.45714286 -0.44285714 -0.42857143 -0.41428571 -0.4 -0.38571429 -0.37142857 -0.35714286 -0.34285714 -0.32857143 -0.31428571 -0.3 -0.28571429 -0.27142857 -0.25714286 -0.24285714 -0.22857143 -0.21428571 -0.2 -0.18571429 -0.17142857 -0.15714286 -0.14285714 -0.12857143 -0.11428571 -0.1 -0.08571429 -0.07142857 -0.05714286 -0.04285714 -0.02857143 -0.01428571 0 0 0 0 0 0
  line L13 (-9.7621, -1.4335) -> (-9.1959, -1.3509)
  arc A27 (-8.0834, -2.0901) -> (-9.1959, -1.3509) centre (-9.0515, -2.3404) ccw
  arc A28 (-8.0834, -2.0901) -> (-8.0454, -2.2316) centre (0, 0) ccw
  arc A29 (-8.6393, -3.428) -> (-8.0454, -2.2316) centre (-9.0091, -2.4989) ccw
  line L14 (-8.6393, -3.428) -> (-9.171, -3.6396)
  spline S14 degree 5 poles (-9.171, -3.6396) (-9.1775, -3.6422) (-9.1905, -3.6476) (-9.2098, -3.6563) (-9.2349, -3.6691) (-9.2656, -3.6867) (-9.2957, -3.7054) (-9.3255, -3.7248) (-9.3552, -3.7446) (-9.3847, -3.7646) (-9.4141, -3.785) (-9.4433, -3.8057) (-9.4723, -3.8269) (-9.501, -3.8487) (-9.5295, -3.871) (-9.5576, -3.8938) (-9.5856, -3.917) (-9.6133, -3.9407) (-9.6409, -3.9646) (-9.6683, -3.9888) (-9.6955, -4.0134) (-9.7226, -4.0383) (-9.7494, -4.0635) (-9.7761, -4.089) (-9.8026, -4.1149) (-9.8289, -4.1411) (-9.855, -4.1677) (-9.8809, -4.1945) (-9.9066, -4.2216) (-9.9322, -4.249) (-9.9576, -4.2766) (-9.9829, -4.3045) (-10.0079, -4.3327) (-10.0328, -4.3612) (-10.0575, -4.3899) (-10.082, -4.4189) (-10.1064, -4.4482) (-10.1306, -4.4777) (-10.1546, -4.5075) (-10.1785, -4.5375) (-10.2021, -4.5677) (-10.2256, -4.5982) (-10.249, -4.6289) (-10.2721, -4.6598) (-10.2951, -4.691) (-10.318, -4.7224) (-10.3406, -4.7541) (-10.3631, -4.7859) (-10.3854, -4.818) (-10.4076, -4.8503) (-10.4296, -4.8828) (-10.4514, -4.9155) (-10.473, -4.9485) (-10.4945, -4.9816) (-10.5158, -5.015) (-10.5369, -5.0485) (-10.5579, -5.0823) (-10.5787, -5.1163) (-10.5993, -5.1504) (-10.6197, -5.1848) (-10.64, -5.2193) (-10.6601, -5.2541) (-10.6801, -5.289) (-10.6998, -5.3242) (-10.7194, -5.3595) (-10.7388, -5.395) (-10.7581, -5.4307) (-10.7772, -5.4665) (-10.7961, -5.5026) (-10.8148, -5.5388) (-10.8334, -5.5752) (-10.8481, -5.6045) (-10.859, -5.6265) (-10.8663, -5.6413) (-10.8699, -5.6486) knots 0 0 0 0 0 0 0.01428571 0.02857143 0.04285714 0.05714286 0.07142857 0.08571429 0.1 0.11428571 0.12857143 0.14285714 0.15714286 0.17142857 0.18571429 0.2 0.21428571 0.22857143 0.24285714 0.25714286 0.27142857 0.28571429 0.3 0.31428571 0.32857143 0.34285714 0.35714286 0.37142857 0.38571429 0.4 0.41428571 0.42857143 0.44285714 0.45714286 0.47142857 0.48571429 0.5 0.51428571 0.52857143 0.54285714 0.55714286 0.57142857 0.58571429 0.6 0.61428571 0.62857143 0.64285714 0.65714286 0.67142857 0.68571429 0.7 0.71428571 0.72857143 0.74285714 0.75714286 0.77142857 0.78571429 0.8 0.81428571 0.82857143 0.84285714 0.85714286 0.87142857 0.88571429 0.9 0.91428571 0.92857143 0.94285714 0.95714286 0.97142857 0.98571429 1 1 1 1 1 1
  arc A30 (-10.8699, -5.6486) -> (-10.3268, -6.5893) centre (0, 0) ccw
  spline S15 degree 5 poles (-10.3268, -6.5893) (-10.3186, -6.5899) (-10.3022, -6.5909) (-10.2777, -6.5925) (-10.245, -6.5944) (-10.2042, -6.5965) (-10.1634, -6.5984) (-10.1228, -6.6) (-10.0821, -6.6014) (-10.0416, -6.6026) (-10.0012, -6.6036) (-9.9608, -6.6042) (-9.9205, -6.6047) (-9.8802, -6.6049) (-9.8401, -6.6049) (-9.8, -6.6046) (-9.76, -6.604) (-9.7202, -6.6033) (-9.6803, -6.6022) (-9.6406, -6.601) (-9.601, -6.5994) (-9.5615, -6.5977) (-9.522, -6.5957) (-9.4827, -6.5934) (-9.4434, -6.5909) (-9.4043, -6.5881) (-9.3652, -6.585) (-9.3263, -6.5818) (-9.2875, -6.5782) (-9.2487, -6.5744) (-9.2101, -6.5703) (-9.1716, -6.566) (-9.1332, -6.5614) (-9.095, -6.5566) (-9.0568, -6.5515) (-9.0188, -6.5461) (-8.9809, -6.5404) (-8.9431, -6.5345) (-8.9054, -6.5283) (-8.8679, -6.5218) (-8.8305, -6.5151) (-8.7933, -6.5081) (-8.7562, -6.5007) (-8.7193, -6.4931) (-8.6825, -6.4852) (-8.6458, -6.4771) (-8.6093, -6.4686) (-8.573, -6.4599) (-8.5368, -6.4508) (-8.5008, -6.4415) (-8.4649, -6.4318) (-8.4293, -6.4218) (-8.3938, -6.4115) (-8.3585, -6.4009) (-8.3235, -6.3899) (-8.2886, -6.3786) (-8.2539, -6.367) (-8.2194, -6.355) (-8.185, -6.3428) (-8.1509, -6.3303) (-8.1171, -6.3173) (-8.0836, -6.3038) (-8.0504, -6.2898) (-8.0175, -6.2753) (-7.9849, -6.2604) (-7.9526, -6.2451) (-7.9205, -6.2295) (-7.8885, -6.2138) (-7.8568, -6.1976) (-7.8255, -6.1809) (-7.795, -6.1631) (-7.7714, -6.1477) (-7.7542, -6.1354) (-7.743, -6.1269) (-7.7374, -6.1225) knots -1 -1 -1 -1 -1 -1 -0.98571429 -0.97142857 -0.95714286 -0.94285714 -0.92857143 -0.91428571 -0.9 -0.88571429 -0.87142857 -0.85714286 -0.84285714 -0.82857143 -0.81428571 -0.8 -0.78571429 -0.77142857 -0.75714286 -0.74285714 -0.72857143 -0.71428571 -0.7 -0.68571429 -0.67142857 -0.65714286 -0.64285714 -0.62857143 -0.61428571 -0.6 -0.58571429 -0.57142857 -0.55714286 -0.54285714 -0.52857143 -0.51428571 -0.5 -0.48571429 -0.47142857 -0.45714286 -0.44285714 -0.42857143 -0.41428571 -0.4 -0.38571429 -0.37142857 -0.35714286 -0.34285714 -0.32857143 -0.31428571 -0.3 -0.28571429 -0.27142857 -0.25714286 -0.24285714 -0.22857143 -0.21428571 -0.2 -0.18571429 -0.17142857 -0.15714286 -0.14285714 -0.12857143 -0.11428571 -0.1 -0.08571429 -0.07142857 -0.05714286 -0.04285714 -0.02857143 -0.01428571 0 0 0 0 0 0
  line L15 (-7.7374, -6.1225) -> (-7.2884, -5.7679)
  arc A31 (-5.9553, -5.8518) -> (-7.2884, -5.7679) centre (-6.6686, -6.5526) ccw
  arc A32 (-5.9553, -5.8518) -> (-5.8518, -5.9553) centre (0, 0) ccw
  arc A33 (-5.7679, -7.2884) -> (-5.8518, -5.9553) centre (-6.5526, -6.6686) ccw
  line L16 (-5.7679, -7.2884) -> (-6.1225, -7.7374)
  spline S16 degree 5 poles (-6.1225, -7.7374) (-6.1269, -7.743) (-6.1354, -7.7542) (-6.1477, -7.7714) (-6.1631, -7.795) (-6.1809, -7.8255) (-6.1976, -7.8568) (-6.2138, -7.8885) (-6.2295, -7.9205) (-6.2451, -7.9526) (-6.2604, -7.9849) (-6.2753, -8.0175) (-6.2898, -8.0504) (-6.3038, -8.0836) (-6.3173, -8.1171) (-6.3303, -8.1509) (-6.3428, -8.185) (-6.355, -8.2194) (-6.367, -8.2539) (-6.3786, -8.2886) (-6.3899, -8.3235) (-6.4009, -8.3585) (-6.4115, -8.3938) (-6.4218, -8.4293) (-6.4318, -8.4649) (-6.4415, -8.5008) (-6.4508, -8.5368) (-6.4599, -8.573) (-6.4686, -8.6093) (-6.4771, -8.6458) (-6.4852, -8.6825) (-6.4931, -8.7193) (-6.5007, -8.7562) (-6.5081, -8.7933) (-6.5151, -8.8305) (-6.5218, -8.8679) (-6.5283, -8.9054) (-6.5345, -8.9431) (-6.5404, -8.9809) (-6.5461, -9.0188) (-6.5515, -9.0568) (-6.5566, -9.095) (-6.5614, -9.1332) (-6.566, -9.1716) (-6.5703, -9.2101) (-6.5744, -9.2487) (-6.5782, -9.2875) (-6.5818, -9.3263) (-6.585, -9.3652) (-6.5881, -9.4043) (-6.5909, -9.4434) (-6.5934, -9.4827) (-6.5957, -9.522) (-6.5977, -9.5615) (-6.5994, -9.601) (-6.601, -9.6406) (-6.6022, -9.6803) (-6.6033, -9.7202) (-6.604, -9.76) (-6.6046, -9.8) (-6.6049, -9.8401) (-6.6049, -9.8802) (-6.6047, -9.9205) (-6.6042, -9.9608) (-6.6036, -10.0012) (-6.6026, -10.0416) (-6.6014, -10.0821) (-6.6, -10.1228) (-6.5984, -10.1634) (-6.5965, -10.2042) (-6.5944, -10.245) (-6.5925, -10.2777) (-6.5909, -10.3022) (-6.5899, -10.3186) (-6.5893, -10.3268) knots 0 0 0 0 0 0 0.01428571 0.02857143 0.04285714 0.05714286 0.07142857 0.08571429 0.1 0.11428571 0.12857143 0.14285714 0.15714286 0.17142857 0.18571429 0.2 0.21428571 0.22857143 0.24285714 0.25714286 0.27142857 0.28571429 0.3 0.31428571 0.32857143 0.34285714 0.35714286 0.37142857 0.38571429 0.4 0.41428571 0.42857143 0.44285714 0.45714286 0.47142857 0.48571429 0.5 0.51428571 0.52857143 0.54285714 0.55714286 0.57142857 0.58571429 0.6 0.61428571 0.62857143 0.64285714 0.65714286 0.67142857 0.68571429 0.7 0.71428571 0.72857143 0.74285714 0.75714286 0.77142857 0.78571429 0.8 0.81428571 0.82857143 0.84285714 0.85714286 0.87142857 0.88571429 0.9 0.91428571 0.92857143 0.94285714 0.95714286 0.97142857 0.98571429 1 1 1 1 1 1
  arc A34 (-6.5893, -10.3268) -> (-5.6486, -10.8699) centre (0, 0) ccw
  spline S17 degree 5 poles (-5.6486, -10.8699) (-5.6413, -10.8663) (-5.6265, -10.859) (-5.6045, -10.8481) (-5.5752, -10.8334) (-5.5388, -10.8148) (-5.5026, -10.7961) (-5.4665, -10.7772) (-5.4307, -10.7581) (-5.395, -10.7388) (-5.3595, -10.7194) (-5.3242, -10.6998) (-5.289, -10.6801) (-5.2541, -10.6601) (-5.2193, -10.64) (-5.1848, -10.6197) (-5.1504, -10.5993) (-5.1163, -10.5787) (-5.0823, -10.5579) (-5.0485, -10.5369) (-5.015, -10.5158) (-4.9816, -10.4945) (-4.9485, -10.473) (-4.9155, -10.4514) (-4.8828, -10.4296) (-4.8503, -10.4076) (-4.818, -10.3854) (-4.7859, -10.3631) (-4.7541, -10.3406) (-4.7224, -10.318) (-4.691, -10.2951) (-4.6598, -10.2721) (-4.6289, -10.249) (-4.5982, -10.2256) (-4.5677, -10.2021) (-4.5375, -10.1785) (-4.5075, -10.1546) (-4.4777, -10.1306) (-4.4482, -10.1064) (-4.4189, -10.082) (-4.3899, -10.0575) (-4.3612, -10.0328) (-4.3327, -10.0079) (-4.3045, -9.9829) (-4.2766, -9.9576) (-4.249, -9.9322) (-4.2216, -9.9066) (-4.1945, -9.8809) (-4.1677, -9.855) (-4.1411, -9.8289) (-4.1149, -9.8026) (-4.089, -9.7761) (-4.0635, -9.7494) (-4.0383, -9.7226) (-4.0134, -9.6955) (-3.9888, -9.6683) (-3.9646, -9.6409) (-3.9407, -9.6133) (-3.917, -9.5856) (-3.8938, -9.5576) (-3.871, -9.5295) (-3.8487, -9.501) (-3.8269, -9.4723) (-3.8057, -9.4433) (-3.785, -9.4141) (-3.7646, -9.3847) (-3.7446, -9.3552) (-3.7248, -9.3255) (-3.7054, -9.2957) (-3.6867, -9.2656) (-3.6691, -9.2349) (-3.6563, -9.2098) (-3.6476, -9.1905) (-3.6422, -9.1775) (-3.6396, -9.171) knots -1 -1 -1 -1 -1 -1 -0.98571429 -0.97142857 -0.95714286 -0.94285714 -0.92857143 -0.91428571 -0.9 -0.88571429 -0.87142857 -0.85714286 -0.84285714 -0.82857143 -0.81428571 -0.8 -0.78571429 -0.77142857 -0.75714286 -0.74285714 -0.72857143 -0.71428571 -0.7 -0.68571429 -0.67142857 -0.65714286 -0.64285714 -0.62857143 -0.61428571 -0.6 -0.58571429 -0.57142857 -0.55714286 -0.54285714 -0.52857143 -0.51428571 -0.5 -0.48571429 -0.47142857 -0.45714286 -0.44285714 -0.42857143 -0.41428571 -0.4 -0.38571429 -0.37142857 -0.35714286 -0.34285714 -0.32857143 -0.31428571 -0.3 -0.28571429 -0.27142857 -0.25714286 -0.24285714 -0.22857143 -0.21428571 -0.2 -0.18571429 -0.17142857 -0.15714286 -0.14285714 -0.12857143 -0.11428571 -0.1 -0.08571429 -0.07142857 -0.05714286 -0.04285714 -0.02857143 -0.01428571 0 0 0 0 0 0
  line L17 (-3.6396, -9.171) -> (-3.428, -8.6393)
  arc A35 (-2.2316, -8.0454) -> (-3.428, -8.6393) centre (-2.4989, -9.0091) ccw
  arc A36 (-2.2316, -8.0454) -> (-2.0901, -8.0834) centre (0, 0) ccw
  arc A37 (-1.3509, -9.1959) -> (-2.0901, -8.0834) centre (-2.3404, -9.0515) ccw
  line L18 (-1.3509, -9.1959) -> (-1.4335, -9.7621)
  spline S18 degree 5 poles (-1.4335, -9.7621) (-1.4345, -9.7691) (-1.4364, -9.783) (-1.4384, -9.8041) (-1.4399, -9.8322) (-1.44, -9.8676) (-1.4389, -9.903) (-1.437, -9.9385) (-1.4347, -9.9741) (-1.4321, -10.0097) (-1.4292, -10.0453) (-1.4258, -10.081) (-1.422, -10.1167) (-1.4175, -10.1525) (-1.4124, -10.1882) (-1.4067, -10.224) (-1.4005, -10.2599) (-1.3939, -10.2957) (-1.387, -10.3316) (-1.3797, -10.3674) (-1.3721, -10.4033) (-1.364, -10.4391) (-1.3556, -10.475) (-1.3469, -10.5109) (-1.3377, -10.5468) (-1.3281, -10.5826) (-1.3182, -10.6185) (-1.3079, -10.6543) (-1.2973, -10.6902) (-1.2864, -10.726) (-1.2752, -10.7619) (-1.2636, -10.7977) (-1.2517, -10.8335) (-1.2395, -10.8693) (-1.227, -10.905) (-1.2141, -10.9408) (-1.2009, -10.9765) (-1.1875, -11.0122) (-1.1737, -11.0479) (-1.1597, -11.0835) (-1.1453, -11.1191) (-1.1307, -11.1547) (-1.1158, -11.1903) (-1.1005, -11.2259) (-1.085, -11.2614) (-1.0692, -11.2968) (-1.0532, -11.3323) (-1.0368, -11.3677) (-1.0202, -11.4031) (-1.0033, -11.4384) (-0.9861, -11.4737) (-0.9687, -11.5089) (-0.951, -11.5441) (-0.933, -11.5793) (-0.9148, -11.6144) (-0.8963, -11.6495) (-0.8775, -11.6845) (-0.8585, -11.7195) (-0.8392, -11.7545) (-0.8197, -11.7894) (-0.7999, -11.8242) (-0.7799, -11.859) (-0.7596, -11.8937) (-0.7391, -11.9284) (-0.7183, -11.963) (-0.6972, -11.9976) (-0.6759, -12.0321) (-0.6544, -12.0666) (-0.6327, -12.101) (-0.6106, -12.1353) (-0.5884, -12.1696) (-0.5704, -12.197) (-0.5568, -12.2175) (-0.5477, -12.2311) (-0.5431, -12.238) knots 0 0 0 0 0 0 0.01428571 0.02857143 0.04285714 0.05714286 0.07142857 0.08571429 0.1 0.11428571 0.12857143 0.14285714 0.15714286 0.17142857 0.18571429 0.2 0.21428571 0.22857143 0.24285714 0.25714286 0.27142857 0.28571429 0.3 0.31428571 0.32857143 0.34285714 0.35714286 0.37142857 0.38571429 0.4 0.41428571 0.42857143 0.44285714 0.45714286 0.47142857 0.48571429 0.5 0.51428571 0.52857143 0.54285714 0.55714286 0.57142857 0.58571429 0.6 0.61428571 0.62857143 0.64285714 0.65714286 0.67142857 0.68571429 0.7 0.71428571 0.72857143 0.74285714 0.75714286 0.77142857 0.78571429 0.8 0.81428571 0.82857143 0.84285714 0.85714286 0.87142857 0.88571429 0.9 0.91428571 0.92857143 0.94285714 0.95714286 0.97142857 0.98571429 1 1 1 1 1 1
  arc A38 (-0.5431, -12.238) -> (0.5431, -12.238) centre (0, 0) ccw
  spline S19 degree 5 poles (0.5431, -12.238) (0.5477, -12.2311) (0.5568, -12.2175) (0.5704, -12.197) (0.5884, -12.1696) (0.6106, -12.1353) (0.6327, -12.101) (0.6544, -12.0666) (0.6759, -12.0321) (0.6972, -11.9976) (0.7183, -11.963) (0.7391, -11.9284) (0.7596, -11.8937) (0.7799, -11.859) (0.7999, -11.8242) (0.8197, -11.7894) (0.8392, -11.7545) (0.8585, -11.7195) (0.8775, -11.6845) (0.8963, -11.6495) (0.9148, -11.6144) (0.933, -11.5793) (0.951, -11.5441) (0.9687, -11.5089) (0.9861, -11.4737) (1.0033, -11.4384) (1.0202, -11.4031) (1.0368, -11.3677) (1.0532, -11.3323) (1.0692, -11.2968) (1.085, -11.2614) (1.1005, -11.2259) (1.1158, -11.1903) (1.1307, -11.1547) (1.1453, -11.1191) (1.1597, -11.0835) (1.1737, -11.0479) (1.1875, -11.0122) (1.2009, -10.9765) (1.2141, -10.9408) (1.227, -10.905) (1.2395, -10.8693) (1.2517, -10.8335) (1.2636, -10.7977) (1.2752, -10.7619) (1.2864, -10.726) (1.2973, -10.6902) (1.3079, -10.6543) (1.3182, -10.6185) (1.3281, -10.5826) (1.3377, -10.5468) (1.3469, -10.5109) (1.3556, -10.475) (1.364, -10.4391) (1.3721, -10.4033) (1.3797, -10.3674) (1.387, -10.3316) (1.3939, -10.2957) (1.4005, -10.2599) (1.4067, -10.224) (1.4124, -10.1882) (1.4175, -10.1525) (1.422, -10.1167) (1.4258, -10.081) (1.4292, -10.0453) (1.4321, -10.0097) (1.4347, -9.9741) (1.437, -9.9385) (1.4389, -9.903) (1.44, -9.8676) (1.4399, -9.8322) (1.4384, -9.8041) (1.4364, -9.783) (1.4345, -9.7691) (1.4335, -9.7621) knots -1 -1 -1 -1 -1 -1 -0.98571429 -0.97142857 -0.95714286 -0.94285714 -0.92857143 -0.91428571 -0.9 -0.88571429 -0.87142857 -0.85714286 -0.84285714 -0.82857143 -0.81428571 -0.8 -0.78571429 -0.77142857 -0.75714286 -0.74285714 -0.72857143 -0.71428571 -0.7 -0.68571429 -0.67142857 -0.65714286 -0.64285714 -0.62857143 -0.61428571 -0.6 -0.58571429 -0.57142857 -0.55714286 -0.54285714 -0.52857143 -0.51428571 -0.5 -0.48571429 -0.47142857 -0.45714286 -0.44285714 -0.42857143 -0.41428571 -0.4 -0.38571429 -0.37142857 -0.35714286 -0.34285714 -0.32857143 -0.31428571 -0.3 -0.28571429 -0.27142857 -0.25714286 -0.24285714 -0.22857143 -0.21428571 -0.2 -0.18571429 -0.17142857 -0.15714286 -0.14285714 -0.12857143 -0.11428571 -0.1 -0.08571429 -0.07142857 -0.05714286 -0.04285714 -0.02857143 -0.01428571 0 0 0 0 0 0
  line L19 (1.4335, -9.7621) -> (1.3509, -9.1959)
  arc A39 (2.0901, -8.0834) -> (1.3509, -9.1959) centre (2.3404, -9.0515) ccw
  arc A40 (2.0901, -8.0834) -> (2.2316, -8.0454) centre (0, 0) ccw
  arc A41 (3.428, -8.6393) -> (2.2316, -8.0454) centre (2.4989, -9.0091) ccw
  line L20 (3.428, -8.6393) -> (3.6396, -9.171)
  spline S20 degree 5 poles (3.6396, -9.171) (3.6422, -9.1775) (3.6476, -9.1905) (3.6563, -9.2098) (3.6691, -9.2349) (3.6867, -9.2656) (3.7054, -9.2957) (3.7248, -9.3255) (3.7446, -9.3552) (3.7646, -9.3847) (3.785, -9.4141) (3.8057, -9.4433) (3.8269, -9.4723) (3.8487, -9.501) (3.871, -9.5295) (3.8938, -9.5576) (3.917, -9.5856) (3.9407, -9.6133) (3.9646, -9.6409) (3.9888, -9.6683) (4.0134, -9.6955) (4.0383, -9.7226) (4.0635, -9.7494) (4.089, -9.7761) (4.1149, -9.8026) (4.1411, -9.8289) (4.1677, -9.855) (4.1945, -9.8809) (4.2216, -9.9066) (4.249, -9.9322) (4.2766, -9.9576) (4.3045, -9.9829) (4.3327, -10.0079) (4.3612, -10.0328) (4.3899, -10.0575) (4.4189, -10.082) (4.4482, -10.1064) (4.4777, -10.1306) (4.5075, -10.1546) (4.5375, -10.1785) (4.5677, -10.2021) (4.5982, -10.2256) (4.6289, -10.249) (4.6598, -10.2721) (4.691, -10.2951) (4.7224, -10.318) (4.7541, -10.3406) (4.7859, -10.3631) (4.818, -10.3854) (4.8503, -10.4076) (4.8828, -10.4296) (4.9155, -10.4514) (4.9485, -10.473) (4.9816, -10.4945) (5.015, -10.5158) (5.0485, -10.5369) (5.0823, -10.5579) (5.1163, -10.5787) (5.1504, -10.5993) (5.1848, -10.6197) (5.2193, -10.64) (5.2541, -10.6601) (5.289, -10.6801) (5.3242, -10.6998) (5.3595, -10.7194) (5.395, -10.7388) (5.4307, -10.7581) (5.4665, -10.7772) (5.5026, -10.7961) (5.5388, -10.8148) (5.5752, -10.8334) (5.6045, -10.8481) (5.6265, -10.859) (5.6413, -10.8663) (5.6486, -10.8699) knots 0 0 0 0 0 0 0.01428571 0.02857143 0.04285714 0.05714286 0.07142857 0.08571429 0.1 0.11428571 0.12857143 0.14285714 0.15714286 0.17142857 0.18571429 0.2 0.21428571 0.22857143 0.24285714 0.25714286 0.27142857 0.28571429 0.3 0.31428571 0.32857143 0.34285714 0.35714286 0.37142857 0.38571429 0.4 0.41428571 0.42857143 0.44285714 0.45714286 0.47142857 0.48571429 0.5 0.51428571 0.52857143 0.54285714 0.55714286 0.57142857 0.58571429 0.6 0.61428571 0.62857143 0.64285714 0.65714286 0.67142857 0.68571429 0.7 0.71428571 0.72857143 0.74285714 0.75714286 0.77142857 0.78571429 0.8 0.81428571 0.82857143 0.84285714 0.85714286 0.87142857 0.88571429 0.9 0.91428571 0.92857143 0.94285714 0.95714286 0.97142857 0.98571429 1 1 1 1 1 1
  arc A42 (5.6486, -10.8699) -> (6.5893, -10.3268) centre (0, 0) ccw